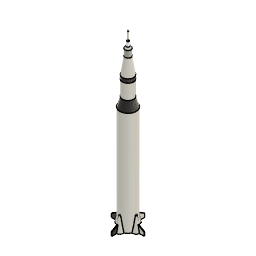
Saturn V Rocket (Autodesk Fusion 360 design; units mm, degrees)
part number: 2026-06-10-19-57-57-392
Autodesk Fusion 360 part; units mm, degrees
sketch "Sketch1" plane through (0, 0, 0) normal (0, 0, 1) x (1, 0, 0)
  circle A0 centre (0, 0) radius 29
  circle A1 centre (0, 0) radius 12
  dimension "d1" = 58
  dimension "d2" = 24
  constraint coincident A0.centre A1.centre
  measures "d1" diameter of A0
  measures "d2" diameter of A1
extrude "Extrude1" add sketch "Sketch1" along normal blind 365
sketch "Sketch5" plane through (0, 0, 365) normal (0, 0, 1) x (-1, 0, 0)
  circle A0 centre (0, 0) radius 12
  circle A1 centre (0, 0) radius 29
extrude "Extrude2" add sketch "Sketch5" along normal blind 32 draft -16 contours A0 | A1
extrude "Extrude3" add 1 faces at (3.304, 5.7227, 397) along direction (0, 0, 1) blind 66
ref_plane "WorkPlane1" through (0, 0, 450) normal (0, 0, 1) x (-1, 0, 0)
split_face "SplitFace1" 1 faces at (19.7995, -0.9882, 441) by plane through (0, 0, 450) normal (0, 0, 1)
extrude "Extrude4" add 1 faces at (3.304, 5.7227, 463) along direction (0, 0, 1) blind 57 draft -9
extrude "Extrude5" add 1 faces at (-3.4389, -1.0607, 520) along direction (0, 0, 1) blind 23
extrude "Extrude6" add 1 faces at (-3.4389, -1.0607, 543) along direction (0, 0, 1) blind 7 draft -35.7
extrude "Extrude7" add 1 faces at (-1.5526, -1.5561, 550) along direction (0, 0, 1) blind 15 draft -6
extrude "Extrude8" add 1 faces at (-1.2859, -1.123, 565) along direction (0, 0, 1) blind 3 draft -30
extrude "Extrude9" add 1 faces at (-0.4946, 0.1457, 568) along direction (0, 0, 1) blind 27
extrude "Extrude10" add 1 faces at (-0.4946, 0.1457, 595) along direction (0, 0, 1) blind 5 draft -25
sketch "Sketch6" plane through (0, 0, 0) normal (0, 0, -1) x (1, 0, 0)
  circle A0 centre (0, 0) radius 12
  circle A1 centre (0, 0) radius 29
  circle A2 centre (29, 0) radius 12.5
  dimension "d24" = 25
  constraint horizontal A0.centre A2.centre
  constraint coincident A1 A2.centre
  measures "d24" diameter of A2
extrude "Extrude11" add sketch "Sketch6" against normal blind 52 draft -11 contours A1 A2 | A1 A2 picked at (24.8269, -2.2787) picked at (32.6561, -3.1961)
fillet "Fillet1" radius 2.9 1 edges at (31.3922, 0, 52)
sketch "Sketch7" plane through (0, 0, 0) normal (0, 1, 0) x (1, 0, 0)
  line L0 (28, -30.5) -> (28, 0)
  line L1 (28, 0) -> (58, 0)
  line L2 (58, 0) -> (58, -12.5)
  line L3 (58, -12.5) -> (28, -30.5)
  dimension "d29" = 30.5
  dimension "d30" = 30
  dimension "d31" = 12.5
  dimension "d32" = 28
  constraint vertical L0
  constraint perpendicular L0 L1
  constraint perpendicular L1 L2
  constraint horizontal origin L0.end
  measures "d29" distance of L0.start L0.end
  measures "d30" distance of L0.end L1.end
  measures "d31" distance of L1.end L2.end
  measures "d32" distance of origin L0
extrude "Extrude12" add sketch "Sketch7" along normal mid plane 2.4
pattern_circular "C-Pattern1" count 4 over 360 about axis through (0, 0, -0.0046) along (0, 0, 1) of "Extrude11", "Fillet1", "Extrude12"
